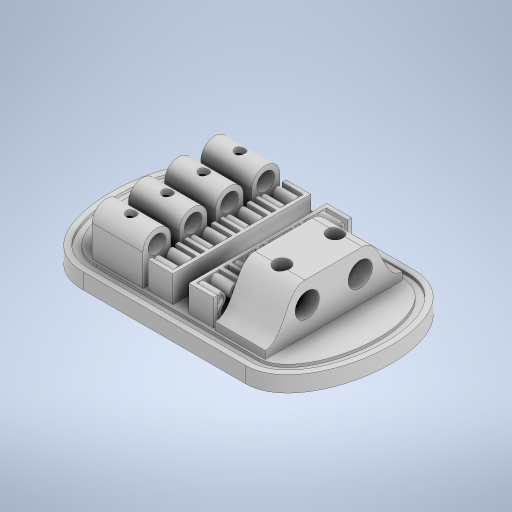
# Autodesk Inventor part: CO-1-01-fuseBox
Saved by Autodesk Inventor 2023 (Build 270158000, 158)
## iProperties
Created: 2023-02-27
Part Number: CO-1-01-fuseBox
Material: Generic
Document SubType Name: Modeling
Designer: t205b
Density: 1 g/cm^3
Appearance: Default
Author: t205b
Autodesk Inventor part; units mm, degrees
sketch "Sketch3" plane through (0, 0, 0) normal (0, 1, 0) x (-1, 0, 0)
  spline S0 degree 3 poles (-36.65, 37.75) (-66.3724, 37.75) (-73.5943, -37.75) (-36.65, -37.75) knots 0 0 0 0 1 1 1 1
  line L0 (-36.65, -37.75) -> (36.65, -37.75)
  line L1 (100, 0) -> (-100, 0)
  line L2 (0, 75) -> (0, -75)
  line L3 (140, 0) -> (-140, 0) projected
  line L4 (0, -105) -> (0, 105) projected
  line L5 (-36.65, 37.75) -> (36.65, 37.75)
  spline S1 degree 4 poles (36.65, 37.75) (64.3582, 37.75) (66.3724, 0) (64.3582, -37.75) (36.65, -37.75) knots 0 0 0 0 0 1 1 1 1 1
  point P0 (0, 0)
  point P1 (-61.65, 0)
  point P2 (0, 0)
  point P3 (61.65, 0)
  dimension "d32" = 200
  dimension "d33" = 150
  dimension "d34" = 75
  dimension "d35" = 100
  dimension "d36" = 37.75
  dimension "d37" = 61.65
  dimension "d38" = 25
  dimension "d39" = 75.5
  dimension "d40" = 25
  constraints: 8 end point, 6 horizontal, 2 collinear, 2 point on line, 2 symmetric about line, 1 midpoint, 1 vertical, 1 vertical alignment, 6 other
  measures "d32" distance of L1.start L1.end
  measures "d33" distance of L2.start L2.end
  measures "d34" distance of point (0, 0) L2.end
  measures "d35" distance of point (0, 0) L1.end
  measures "d36" distance between parallel lines of L1 L0
  measures "d37" distance from line of L2 point (-61.65, 0)
  measures "d38" horizontal distance of point (-61.65, 0) L0.start
  measures "d39" distance between parallel lines of L5 L0
  measures "d40" horizontal distance of L0.end point (61.65, 0)
extrude "Extrusion2" add sketch "Sketch3" along normal blind 7.2
sketch "Sketch4" plane through (0, 7.2, 0) normal (0, 1, 0) x (1, 0, 0)
  line L0 (-36.65, -37.75) -> (36.65, -37.75) projected
  spline S0 degree 3 poles (36.65, -37.75) (66.3724, -37.75) (73.5943, 37.75) (36.65, 37.75) knots 0 0 0 0 1 1 1 1
  line L1 (36.65, 37.75) -> (-36.65, 37.75) projected
  spline S1 degree 4 poles (-36.65, 37.75) (-64.3582, 37.75) (-66.3724, 0) (-64.3582, -37.75) (-36.65, -37.75) knots 0 0 0 0 0 1 1 1 1 1
  line L2 (36.65, -35.15) -> (-36.65, -35.15)
  line L3 (-36.65, 35.15) -> (36.65, 35.15)
  line L4 (36.65, -32) -> (-36.65, -32)
  line L5 (-36.65, 32) -> (36.65, 32)
  spline S2 degree 5 poles (-36.65, -35.15) (-38.7951, -35.149) (-40.9355, -34.9184) (-43.0555, -34.3853) (-46.9479, -32.645) (-50.1237, -29.806) (-51.4679, -28.2094) (-53.9958, -24.4798) (-55.7766, -20.3315) (-56.5612, -18.0325) (-57.9028, -13.0968) (-58.6606, -8.0384) (-58.9204, -5.3645) (-59.1796, 0) (-58.9204, 5.3645) (-58.6606, 8.0384) (-57.9028, 13.0968) (-56.5612, 18.0325) (-55.7766, 20.3315) (-53.9958, 24.4798) (-51.4679, 28.2094) (-50.1237, 29.806) (-46.9479, 32.645) (-43.0555, 34.3853) (-40.9355, 34.9184) (-38.7951, 35.149) (-36.65, 35.15) knots 0 0 0 0 0 0 0.11508 0.11508 0.11508 0.225967 0.225967 0.225967 0.356046 0.356046 0.356046 0.5 0.5 0.5 0.643954 0.643954 0.643954 0.774033 0.774033 0.774033 0.88492 0.88492 0.88492 1 1 1 1 1 1
  spline S3 degree 5 poles (36.65, 35.15) (38.8444, 35.1493) (41.0355, 34.9067) (43.1996, 34.3601) (47.1853, 32.6249) (50.4881, 29.804) (51.8967, 28.2119) (54.5079, 24.5102) (56.327, 20.3525) (57.1025, 18.0646) (58.3839, 13.1497) (59.0001, 8.107) (59.1641, 5.4459) (59.1963, 0.0809) (58.6482, -5.2565) (58.23, -7.9258) (57.1472, -13.0057) (55.486, -17.9261) (54.5457, -20.2359) (52.5203, -24.3703) (49.8538, -28.1181) (48.4863, -29.7243) (45.5873, -32.4365) (42.0779, -34.2692) (40.3126, -34.8729) (38.479, -35.1493) (36.65, -35.15) knots 0 0 0 0 0 0 0.118721 0.118721 0.118721 0.23255 0.23255 0.23255 0.362852 0.362852 0.362852 0.506829 0.506829 0.506829 0.652778 0.652778 0.652778 0.787419 0.787419 0.787419 0.900976 0.900976 0.900976 1 1 1 1 1 1
  spline S4 degree 5 poles (-36.65, -32) (-38.4313, -31.9991) (-40.2071, -31.8168) (-41.973, -31.3923) (-45.254, -29.9388) (-47.9096, -27.5288) (-49.0424, -26.1594) (-51.279, -22.8321) (-52.852, -19.1329) (-53.5716, -17.0114) (-54.8234, -12.3836) (-55.5313, -7.642) (-55.7772, -5.0998) (-56.0228, 0) (-55.7772, 5.0998) (-55.5313, 7.642) (-54.8234, 12.3836) (-53.5716, 17.0114) (-52.852, 19.1329) (-51.279, 22.8321) (-49.0424, 26.1594) (-47.9096, 27.5288) (-45.254, 29.9388) (-41.973, 31.3923) (-40.2071, 31.8168) (-38.4313, 31.9991) (-36.65, 32) knots 0 0 0 0 0 0 0.106905 0.106905 0.106905 0.21262 0.21262 0.21262 0.346882 0.346882 0.346882 0.5 0.5 0.5 0.653118 0.653118 0.653118 0.78738 0.78738 0.78738 0.893095 0.893095 0.893095 1 1 1 1 1 1
  spline S5 degree 5 poles (36.65, 32) (38.4906, 31.9993) (40.3274, 31.8039) (42.1467, 31.3587) (45.524, 29.8989) (48.3077, 27.4963) (49.5, 26.1293) (51.8011, 22.8434) (53.4009, 19.1536) (54.1048, 17.0615) (55.2895, 12.4921) (55.8589, 7.8049) (56.0122, 5.2946) (56.041, 0.221) (55.523, -4.8266) (55.127, -7.3572) (54.1106, -12.1313) (52.5533, -16.7561) (51.6809, -18.9069) (49.8554, -22.6513) (47.4533, -26.0492) (46.267, -27.4584) (43.8621, -29.7468) (40.9405, -31.2919) (39.5479, -31.7812) (38.0961, -31.9994) (36.65, -32) knots 0 0 0 0 0 0 0.111514 0.111514 0.111514 0.220328 0.220328 0.220328 0.353718 0.353718 0.353718 0.505824 0.505824 0.505824 0.66079 0.66079 0.66079 0.801131 0.801131 0.801131 0.912291 0.912291 0.912291 1 1 1 1 1 1
  point P0 (0, 0)
  dimension "d43" = 2.6
  dimension "d44" = 5.75
  constraints: 8 end point, 6 parallel, 6 vertical alignment, 8 other
  measures "d43" distance between parallel lines of L0 L2
  measures "d44" distance between parallel lines of L0 L4
ref_plane "Work Plane1" through (38.75, 0, 0) normal (1, 0, 0) x (0, 1, 0)
sketch "Sketch5" plane through (38.75, 0, 0) normal (1, 0, 0) x (0, 1, 0)
  line L0 (29.3, 13) -> (29.3, -13)
  line L1 (7.2, 31) -> (10.7, 31)
  line L2 (7.2, -31) -> (10.7, -31)
  line L3 (10.7, 31) -> (10.7, 22) construction
  line L4 (10.7, 22) -> (29.3, 22) construction
  line L5 (29.3, 22) -> (29.3, 13) construction
  spline S0 degree 3 poles (10.7, 31) (10.7, 22) (29.3, 22) (29.3, 13) knots 1 1 1 1 2 2 2 2
  line L6 (10.7, -31) -> (10.7, -22) construction
  line L7 (10.7, -22) -> (29.3, -22) construction
  line L8 (29.3, -22) -> (29.3, -13) construction
  spline S1 degree 3 poles (10.7, -31) (10.7, -22) (29.3, -22) (29.3, -13) knots 1 1 1 1 2 2 2 2
  line L9 (7.2, 31) -> (7.2, -31)
  line L10 (7.2, 37.75) -> (7.2, -37.75) projected
  line L11 (-6.2242, 0) -> (37.3454, 0) projected
  circle A0 centre (19.125, 12) radius 5.425
  circle A1 centre (19.125, -12) radius 5.425
  point P0 (0, 0)
  dimension "d46" = 22.1
  dimension "d47" = 62
  dimension "d48" = 31
  dimension "d49" = 3.5
  dimension "d51" = 26
  dimension "d52" = 13
  dimension "d53" = 10.85
  dimension "d54" = 12
  dimension "d55" = 12
  dimension "d56" = 10.175
  dimension "d57" = 10.175
  constraints: 8 end point, 6 vertical, 4 horizontal, 3 parallel, 2 centre point, 1 collinear, 1 equal radius, 6 other
  measures "d46" distance between parallel lines of L0 L9
  measures "d47" distance between parallel lines of L2 L1
  measures "d48" distance between parallel lines of L11 L2
  measures "d49" distance of L2.start L2.end
  measures "d51" distance of L0.start L0.end
  measures "d52" distance from line of L11 L0.end
  measures "d53" diameter of A1
  measures "d54" distance from line of L11 A1.centre
  measures "d55" distance from line of L11 A0.centre
  measures "d56" distance from line of L0 A1.centre
  measures "d57" distance from line of L0 A0.centre
extrude "Extrusion3" cut sketch "Sketch4" against normal blind 1.25 contours L2 S2 L3 S3
extrude "Extrusion4" add sketch "Sketch5" against normal blind 22.68
sketch "Sketch6" plane through (38.75, 29.3, 13) normal (0, 1, 0) x (1, 0, 0)
  line L0 (-22.68, -4.425) -> (-22.68, 6.425) projected
  line L1 (0, 6.425) -> (0, -4.425) projected
  line L2 (-22.68, 19.575) -> (-22.68, 30.425) projected
  line L3 (0, 30.425) -> (0, 19.575) projected
  line L4 (0, -18) -> (-22.68, -18) construction
  line L5 (-11.34, -18) -> (-11.34, 44) construction
  line L6 (-22.68, 44) -> (0, 44) construction
  line L7 (-22.68, -18) -> (-22.68, 44) construction
  line L8 (-22.68, 1) -> (0, 1) construction
  line L9 (0, 44) -> (0, -18) construction
  line L10 (-22.68, 25) -> (0, 25) construction
  circle A0 centre (-11.34, 1) radius 3.5
  circle A1 centre (-11.34, 25) radius 3.5
  point P0 (-38.75, 13)
  dimension "d62" = 7
  dimension "d63" = 7
  constraints: 7 midpoint, 6 end point, 3 point on line, 2 centre point, 1 perpendicular
  measures "d62" diameter of A0
  measures "d63" diameter of A1
extrude "Extrusion5" cut sketch "Sketch6" against normal blind 7
ref_plane "Work Plane2" through (-16.68, 0, 0) normal (-1, 0, 0) x (0, 0, 1)
sketch "Sketch7" plane through (-16.68, 0, 0) normal (-1, 0, 0) x (0, 0, 1)
  line L0 (-31, 10.7) -> (-31, 7.2) projected
  line L1 (-31, 7.2) -> (-31, 21.375)
  line L2 (-31, 7.2) -> (31, 7.2) projected
  line L3 (-18.35, 7.2) -> (-18.35, 21.375)
  arc A0 (-18.35, 21.375) -> (-31, 21.375) centre (-24.675, 21.375) ccw
  circle A1 centre (-24.675, 21.375) radius 4
  line L4 (-14.6, 7.2) -> (-14.6, 21.375)
  arc A2 (-1.95, 21.375) -> (-14.6, 21.375) centre (-8.275, 21.375) ccw
  circle A3 centre (-8.275, 21.375) radius 4
  line L5 (-1.95, 7.2) -> (-1.95, 21.375)
  line L6 (1.8, 7.2) -> (1.8, 21.375)
  arc A4 (14.45, 21.375) -> (1.8, 21.375) centre (8.125, 21.375) ccw
  circle A5 centre (8.125, 21.375) radius 4
  line L7 (14.45, 7.2) -> (14.45, 21.375)
  line L8 (18.2, 7.2) -> (18.2, 21.375)
  arc A6 (30.85, 21.375) -> (18.2, 21.375) centre (24.525, 21.375) ccw
  circle A7 centre (24.525, 21.375) radius 4
  line L9 (30.85, 7.2) -> (30.85, 21.375)
  point P0 (0, 0)
  point P1 (-31, 14.2875)
  point P2 (-14.6, 14.2875)
  point P3 (1.8, 14.2875)
  point P4 (18.2, 14.2875)
  dimension "d67" = 12.65
  dimension "d69" = 14.175
  dimension "d70" = 8
  dimension "d73" = 16.4
  constraints: 16 end point, 8 centre point, 8 point on circle, 4 coincident, 2 tangent, 2 vertical, 1 horizontal, 1 midpoint, 1 point on line, 33 other
  measures "d67" distance from line of point (-31, 14.288) L3
  measures "d69" distance from line of L2 A0.centre
  measures "d70" diameter of A1
  measures "d73" distance of L0.end L4.start
extrude "Extrusion6" add sketch "Sketch7" along normal blind 23
ref_plane "Work Plane3" through (0, 27.5, 0) normal (0, 1, 0) x (1, 0, 0)
sketch "Sketch8" plane through (0, 27.5, 0) normal (0, 1, 0) x (1, 0, 0)
  circle A0 centre (-28.23, 24.675) radius 2.2
  line L0 (-39.68, 20.675) -> (-39.68, 28.675) projected
  line L1 (-16.68, 18.35) -> (-39.68, 18.35) projected
  circle A1 centre (-28.23, 8.275) radius 2.2
  circle A2 centre (-28.23, -8.125) radius 2.2
  circle A3 centre (-28.23, -24.525) radius 2.2
  line L2 (-39.68, -28.525) -> (-39.68, -20.525) projected
  point P0 (0, 0)
  point P1 (-28.18, 18.35)
  dimension "d81" = 4.4
  dimension "d82" = 11.45
  dimension "d84" = 8
  dimension "d85" = 4
  dimension "d88" = 16.4
  constraints: 4 centre point, 1 midpoint, 1 vertical, 6 other
  measures "d81" diameter of A0
  measures "d82" distance from line of L0 A0.centre
  measures "d84" distance of L0.start L0.end
  measures "d85" vertical distance of A0.centre L0.start
  measures "d88" distance of A0.centre A1.centre
extrude "Extrusion7" cut sketch "Sketch8" along normal mid plane 6
sketch "Sketch9" plane through (0, 7.2, 0) normal (0, 1, 0) x (1, 0, 0)
  line L0 (14.87, -30.35) -> (3.62, -30.35)
  line L1 (3.62, -30.35) -> (3.62, 32.05)
  line L2 (3.62, 32.05) -> (14.87, 32.05)
  line L3 (36.65, 32) -> (-36.65, 32) projected
  line L4 (14.87, 32.05) -> (14.87, 30.25)
  line L5 (14.87, 30.25) -> (5.22, 30.25)
  line L6 (5.22, 30.25) -> (5.22, 19.75)
  line L7 (5.22, 19.75) -> (14.87, 19.75)
  line L8 (14.87, 19.75) -> (14.87, 17.95)
  line L9 (14.87, 17.95) -> (5.22, 17.95)
  line L10 (5.22, 17.95) -> (5.22, 15.95)
  line L11 (5.22, 15.95) -> (14.87, 15.95)
  line L12 (14.87, 15.95) -> (14.87, 14.15)
  line L13 (14.87, 14.15) -> (5.22, 14.15)
  line L14 (5.22, 14.15) -> (5.22, 3.65)
  line L15 (5.22, 3.65) -> (14.87, 3.65)
  line L16 (14.87, 3.65) -> (14.87, 1.85)
  line L17 (14.87, 1.85) -> (5.22, 1.85)
  line L18 (5.22, 1.85) -> (5.22, -0.15)
  line L19 (5.22, -0.15) -> (14.87, -0.15)
  line L20 (14.87, -0.15) -> (14.87, -1.95)
  line L21 (14.87, -1.95) -> (5.22, -1.95)
  line L22 (5.22, -1.95) -> (5.22, -12.45)
  line L23 (5.22, -12.45) -> (14.87, -12.45)
  line L24 (14.87, -12.45) -> (14.87, -14.25)
  line L25 (14.87, -14.25) -> (5.22, -14.25)
  line L26 (14.87, -30.35) -> (14.87, -28.55)
  line L27 (14.87, -28.55) -> (5.22, -28.55)
  line L28 (5.22, -28.55) -> (5.22, -18.05)
  line L29 (5.22, -18.05) -> (14.87, -18.05)
  line L30 (14.87, -18.05) -> (14.87, -16.25)
  line L31 (14.87, -16.25) -> (5.22, -16.25)
  line L32 (5.22, -16.25) -> (5.22, -14.25)
  line L33 (-36.65, -37.75) -> (36.65, -37.75) projected
  line L34 (16.07, -31) -> (16.07, 31) projected
  point P0 (0, 0)
  dimension "d96" = 1.8
  dimension "d97" = 10.5
  dimension "d99" = 2
  dimension "d100" = 7.4
  dimension "d101" = 1.2
  dimension "d102" = 11.25
  dimension "d103" = 1.6
  dimension "d104" = 9.65
  constraints: 64 end point, 21 perpendicular, 15 equal length, 15 point on line, 3 vertical, 1 horizontal, 1 parallel
  measures "d96" distance of L2.end L4.end
  measures "d97" distance of L5.end L6.end
  measures "d99" distance of L9.end L10.end
  measures "d100" distance between parallel lines of L0 L33
  measures "d101" distance between parallel lines of L34 L26
  measures "d102" distance of L0.start L0.end
  measures "d103" distance between parallel lines of L1 L28
  measures "d104" distance of L28.end L29.end
extrude "Extrusion8" add sketch "Sketch9" along normal blind 12
mirror "Mirror1" about plane through (0, 0, 0) normal (1, 0, 0) of "Extrusion8"
sketch "Sketch10" plane through (5.22, 7.2, -19.75) normal (1, 0, 0) x (0, 0, -1)
  spline S0 degree 4 poles (9.425, 7.8) (9.2346, 15.5874) (3.5799, 6.3679) (8.4396, 8.6805) (9.5353, 0.0883) (0.3147, 0.0883) (1.4104, 8.6805) (6.2701, 6.3679) (0.6154, 15.5874) (0.425, 7.8) knots 0 0 0 0 0 0.26738 0.381915 0.5 0.618085 0.73262 1 1 1 1 1
  line L0 (18, -7.2) -> (-57.5, -7.2) projected
  circle A0 centre (4.925, 14.175) radius 4 projected
  line L1 (10.5, 0) -> (10.5, 12) projected
  line L2 (0, 0) -> (0, 12) projected
  spline S1 degree 5 poles (9.9249, 7.8122) (9.9112, 8.3424) (9.8831, 8.8754) (9.8254, 9.4003) (9.6956, 10.2438) (9.3803, 11.0296) (9.233, 11.3105) (8.8447, 11.7572) (8.2849, 11.9289) (8.0172, 11.9254) (7.5499, 11.7927) (7.1572, 11.5101) (6.9913, 11.3552) (6.6866, 11.0187) (6.4376, 10.6387) (6.3248, 10.4411) (6.1283, 10.0415) (5.9805, 9.6217) (5.9206, 9.4124) (5.832, 9.0043) (5.8023, 8.5879) (5.8032, 8.3877) (5.8388, 8.0043) (5.9426, 7.634) (6.0089, 7.4611) (6.1664, 7.143) (6.3707, 6.853) (6.4774, 6.7205) (6.6955, 6.473) (6.9228, 6.2339) (7.0324, 6.1174) (7.2492, 5.8753) (7.4479, 5.6181) (7.5423, 5.4826) (7.7229, 5.1905) (7.8675, 4.8789) (7.9319, 4.7123) (8.0408, 4.3629) (8.0994, 4.0015) (8.1154, 3.8144) (8.1173, 3.4409) (8.0532, 3.0731) (8.0035, 2.8936) (7.8624, 2.5396) (7.6466, 2.2251) (7.518, 2.0776) (7.2077, 1.7895) (6.8448, 1.5698) (6.6387, 1.4707) (6.1823, 1.2955) (5.7036, 1.1939) (5.4451, 1.1586) (4.925, 1.1234) (4.4049, 1.1586) (4.1464, 1.1939) (3.6677, 1.2955) (3.2113, 1.4707) (3.0052, 1.5698) (2.6423, 1.7895) (2.332, 2.0776) (2.2034, 2.2251) (1.9876, 2.5396) (1.8465, 2.8936) (1.7968, 3.0731) (1.7327, 3.4409) (1.7346, 3.8144) (1.7506, 4.0015) (1.8092, 4.3629) (1.9181, 4.7123) (1.9825, 4.8789) (2.1271, 5.1905) (2.3077, 5.4826) (2.4021, 5.6181) (2.6008, 5.8753) (2.8176, 6.1174) (2.9272, 6.2339) (3.1545, 6.473) (3.3726, 6.7205) (3.4793, 6.853) (3.6836, 7.143) (3.8411, 7.4611) (3.9074, 7.634) (4.0112, 8.0043) (4.0468, 8.3877) (4.0477, 8.5879) (4.018, 9.0043) (3.9294, 9.4124) (3.8695, 9.6217) (3.7217, 10.0415) (3.5252, 10.4411) (3.4124, 10.6387) (3.1634, 11.0187) (2.8587, 11.3552) (2.6928, 11.5101) (2.3001, 11.7927) (1.8328, 11.9254) (1.5651, 11.9289) (1.0053, 11.7572) (0.617, 11.3105) (0.4697, 11.0296) (0.1544, 10.2438) (0.0246, 9.4003) (-0.0331, 8.8754) (-0.0612, 8.3424) (-0.0749, 7.8122) knots 0 0 0 0 0 0 0.068516 0.068516 0.068516 0.108925 0.108925 0.108925 0.141412 0.141412 0.141412 0.170512 0.170512 0.170512 0.199827 0.199827 0.199827 0.227844 0.227844 0.227844 0.253557 0.253557 0.253557 0.277287 0.277287 0.277287 0.299199 0.299199 0.299199 0.31984 0.31984 0.31984 0.341106 0.341106 0.341106 0.364074 0.364074 0.364074 0.388214 0.388214 0.388214 0.412061 0.412061 0.412061 0.437092 0.437092 0.437092 0.466447 0.466447 0.466447 0.5 0.5 0.5 0.533553 0.533553 0.533553 0.562908 0.562908 0.562908 0.587939 0.587939 0.587939 0.611786 0.611786 0.611786 0.635926 0.635926 0.635926 0.658894 0.658894 0.658894 0.68016 0.68016 0.68016 0.700801 0.700801 0.700801 0.722713 0.722713 0.722713 0.746443 0.746443 0.746443 0.772156 0.772156 0.772156 0.800173 0.800173 0.800173 0.829488 0.829488 0.829488 0.858588 0.858588 0.858588 0.891075 0.891075 0.891075 0.931484 0.931484 0.931484 1 1 1 1 1 1
  spline S2 degree 5 poles (8.9251, 7.7878) (8.9156, 8.1863) (8.8951, 8.5845) (8.862, 8.982) (8.7864, 9.5781) (8.6369, 10.1595) (8.5726, 10.3494) (8.4781, 10.5939) (8.3163, 10.7986) (8.2781, 10.8377) (8.1878, 10.9138) (8.0751, 10.8858) (8.0329, 10.8704) (7.8948, 10.8043) (7.7769, 10.7091) (7.7001, 10.6385) (7.5384, 10.4662) (7.3981, 10.2754) (7.3256, 10.1643) (7.1896, 9.9331) (7.076, 9.6902) (7.0241, 9.565) (6.9367, 9.3229) (6.8726, 9.0735) (6.848, 8.9541) (6.8146, 8.7326) (6.8071, 8.5088) (6.8097, 8.4067) (6.8275, 8.2172) (6.872, 8.0324) (6.8987, 7.9482) (6.9658, 7.7815) (7.0552, 7.6255) (7.1058, 7.5492) (7.2257, 7.386) (7.3586, 7.233) (7.4336, 7.1511) (7.6023, 6.9707) (7.7708, 6.7903) (7.8622, 6.6896) (8.0538, 6.4687) (8.2324, 6.2371) (8.3234, 6.1097) (8.5042, 5.834) (8.6602, 5.5436) (8.7347, 5.3872) (8.8735, 5.0555) (8.9774, 4.7111) (9.0214, 4.5298) (9.0913, 4.1524) (9.1162, 3.7693) (9.1167, 3.5718) (9.091, 3.1693) (9.0079, 2.7746) (8.9499, 2.5766) (8.7993, 2.1842) (8.5857, 1.8222) (8.4611, 1.6475) (8.1767, 1.3127) (7.8413, 1.0287) (7.6582, 0.8975) (7.2631, 0.6563) (6.8378, 0.4729) (6.6134, 0.3934) (6.1464, 0.2593) (5.6669, 0.1807) (5.4202, 0.1542) (4.925, 0.1278) (4.4298, 0.1542) (4.1831, 0.1807) (3.7036, 0.2593) (3.2366, 0.3934) (3.0122, 0.4729) (2.5869, 0.6563) (2.1918, 0.8975) (2.0087, 1.0287) (1.6733, 1.3127) (1.3889, 1.6475) (1.2643, 1.8222) (1.0507, 2.1842) (0.9001, 2.5766) (0.8421, 2.7746) (0.759, 3.1693) (0.7333, 3.5718) (0.7338, 3.7693) (0.7587, 4.1524) (0.8286, 4.5298) (0.8726, 4.7111) (0.9765, 5.0555) (1.1153, 5.3872) (1.1898, 5.5436) (1.3458, 5.834) (1.5266, 6.1097) (1.6176, 6.2371) (1.7962, 6.4687) (1.9878, 6.6896) (2.0792, 6.7903) (2.2477, 6.9707) (2.4164, 7.1511) (2.4914, 7.233) (2.6243, 7.386) (2.7442, 7.5492) (2.7948, 7.6255) (2.8842, 7.7815) (2.9513, 7.9482) (2.978, 8.0324) (3.0225, 8.2172) (3.0403, 8.4067) (3.0429, 8.5088) (3.0354, 8.7326) (3.002, 8.9541) (2.9774, 9.0735) (2.9133, 9.3229) (2.8259, 9.565) (2.774, 9.6902) (2.6604, 9.9331) (2.5244, 10.1643) (2.4519, 10.2754) (2.3116, 10.4662) (2.1499, 10.6385) (2.0731, 10.7091) (1.9552, 10.8043) (1.8171, 10.8704) (1.7749, 10.8858) (1.6622, 10.9138) (1.5719, 10.8377) (1.5337, 10.7986) (1.3719, 10.5939) (1.2774, 10.3494) (1.2131, 10.1595) (1.0636, 9.5781) (0.988, 8.982) (0.9549, 8.5845) (0.9344, 8.1863) (0.9249, 7.7878) knots 0 0 0 0 0 0 0.055885 0.055885 0.055885 0.084022 0.084022 0.084022 0.092088 0.092088 0.092088 0.098739 0.098739 0.098739 0.11327 0.11327 0.11327 0.131845 0.131845 0.131845 0.150825 0.150825 0.150825 0.167895 0.167895 0.167895 0.182171 0.182171 0.182171 0.194496 0.194496 0.194496 0.207309 0.207309 0.207309 0.222875 0.222875 0.222875 0.241932 0.241932 0.241932 0.263859 0.263859 0.263859 0.288106 0.288106 0.288106 0.314213 0.314213 0.314213 0.341823 0.341823 0.341823 0.370614 0.370614 0.370614 0.400541 0.400541 0.400541 0.431996 0.431996 0.431996 0.465289 0.465289 0.465289 0.5 0.5 0.5 0.534711 0.534711 0.534711 0.568004 0.568004 0.568004 0.599459 0.599459 0.599459 0.629386 0.629386 0.629386 0.658177 0.658177 0.658177 0.685787 0.685787 0.685787 0.711894 0.711894 0.711894 0.736141 0.736141 0.736141 0.758068 0.758068 0.758068 0.777125 0.777125 0.777125 0.792691 0.792691 0.792691 0.805504 0.805504 0.805504 0.817829 0.817829 0.817829 0.832105 0.832105 0.832105 0.849175 0.849175 0.849175 0.868155 0.868155 0.868155 0.88673 0.88673 0.88673 0.901261 0.901261 0.901261 0.907912 0.907912 0.907912 0.915978 0.915978 0.915978 0.944115 0.944115 0.944115 1 1 1 1 1 1
  point P0 (-19.75, -7.2)
  point P1 (7.175, 10.8)
  point P2 (6.425, 7.8)
  point P3 (7.925, 5.8)
  point P4 (7.925, 1.8)
  point P5 (1.925, 1.8)
  point P6 (1.925, 5.8)
  point P7 (3.425, 7.8)
  point P8 (2.675, 10.8)
  dimension "d145" = 0.5
  dimension "d146" = 0.5
  dimension "d107" = 9
  dimension "d108" = 3
  dimension "d109" = 6
  dimension "d110" = 3
  dimension "d111" = 1.5
  dimension "d113" = 4.5
  dimension "d114" = 6
  dimension "d115" = 3
  dimension "d116" = 4.5
  dimension "d117" = 2.25
  dimension "d128" = 9
  dimension "d131" = 3
  dimension "d132" = 2
  dimension "d134" = 9
  constraints: 8 horizontal alignment, 14 other
  measures "d107" distance from line of point (7.925, 1.8) L0
  measures "d108" distance of point (6.425, 7.8) point (3.425, 7.8)
  measures "d109" distance of point (1.925, 5.8) point (7.925, 5.8)
  measures "d110" horizontal distance of point (7.925, 5.8) A0.centre
  measures "d111" horizontal distance of A0.centre point (6.425, 7.8)
  measures "d113" horizontal distance of point (9.425, 7.8) A0.centre
  measures "d114" distance of point (1.925, 1.8) point (7.925, 1.8)
  measures "d115" horizontal distance of point (7.925, 1.8) A0.centre
  measures "d116" distance of point (2.675, 10.8) point (7.175, 10.8)
  measures "d117" horizontal distance of point (7.175, 10.8) A0.centre
  measures "d128" vertical distance of point (7.175, 10.8) point (7.925, 1.8)
  measures "d131" vertical distance of point (9.425, 7.8) point (7.175, 10.8)
  measures "d132" vertical distance of point (6.425, 7.8) point (7.925, 5.8)
  measures "d134" distance of point (0.425, 7.8) point (9.425, 7.8)
sketch "Sketch11" plane through (5.22, 7.2, -19.75) normal (1, 0, 0) x (0, 0, -1)
  spline S0 degree 3 poles (8.9251, 7.7878) (8.9155, 8.182) (8.8741, 8.8814) (8.7781, 9.5528) (8.671, 10.0317) (8.591, 10.2839) (8.5088, 10.4858) (8.454, 10.5957) (8.3882, 10.7043) (8.3392, 10.7691) (8.2908, 10.8204) (8.2632, 10.8441) (8.2394, 10.8612) (8.2254, 10.8698) (8.21, 10.8778) (8.1991, 10.8824) (8.1867, 10.8866) (8.1774, 10.889) (8.1656, 10.891) (8.1557, 10.892) (8.1421, 10.8924) (8.13, 10.8919) (8.1093, 10.8895) (8.0851, 10.8848) (8.0419, 10.8717) (7.9966, 10.8526) (7.9205, 10.8115) (7.8352, 10.7535) (7.6994, 10.6366) (7.5755, 10.5043) (7.4257, 10.3122) (7.3122, 10.1409) (7.1833, 9.9132) (7.0917, 9.7231) (6.9941, 9.4824) (6.9303, 9.2898) (6.8694, 9.0545) (6.8358, 8.8724) (6.8124, 8.656) (6.8083, 8.4929) (6.8198, 8.3029) (6.8418, 8.1619) (6.8838, 7.9974) (6.9286, 7.8738) (6.9989, 7.7251) (7.0671, 7.6091) (7.1886, 7.4344) (7.3365, 7.2561) (7.6068, 6.9651) (7.8875, 6.6675) (8.2098, 6.2718) (8.4177, 5.971) (8.6086, 5.6398) (8.7255, 5.4039) (8.8546, 5.0912) (8.9426, 4.8274) (9.0294, 4.4828) (9.0789, 4.1963) (9.1117, 3.8278) (9.113, 3.5263) (9.0789, 3.1453) (9.0211, 2.8396) (8.9069, 2.4636) (8.7812, 2.1705) (8.5805, 1.821) (8.3855, 1.5576) (8.1014, 1.2546) (7.8436, 1.0351) (7.4877, 0.7924) (7.1781, 0.6245) (6.7655, 0.449) (6.417, 0.3363) (5.9641, 0.2305) (5.5906, 0.174) (5.1162, 0.1387) (4.7338, 0.1387) (4.2594, 0.174) (3.8859, 0.2305) (3.433, 0.3363) (3.0845, 0.449) (2.6719, 0.6245) (2.3623, 0.7924) (2.0064, 1.0351) (1.7486, 1.2546) (1.4645, 1.5576) (1.2695, 1.821) (1.0688, 2.1705) (0.9431, 2.4636) (0.8289, 2.8396) (0.7711, 3.1453) (0.737, 3.5263) (0.7383, 3.8278) (0.7711, 4.1963) (0.8206, 4.4828) (0.9074, 4.8274) (0.9954, 5.0912) (1.1245, 5.4039) (1.2414, 5.6398) (1.4323, 5.971) (1.6402, 6.2718) (1.9625, 6.6675) (2.2432, 6.9651) (2.5135, 7.2561) (2.6614, 7.4344) (2.7829, 7.6091) (2.8511, 7.7251) (2.9214, 7.8738) (2.9662, 7.9974) (3.0082, 8.1619) (3.0302, 8.3029) (3.0417, 8.4929) (3.0376, 8.656) (3.0142, 8.8724) (2.9806, 9.0545) (2.9197, 9.2898) (2.8559, 9.4824) (2.7583, 9.7231) (2.6667, 9.9132) (2.5378, 10.1409) (2.4243, 10.3122) (2.2745, 10.5043) (2.1506, 10.6366) (2.0148, 10.7535) (1.9295, 10.8115) (1.8534, 10.8526) (1.8081, 10.8717) (1.7649, 10.8848) (1.7407, 10.8895) (1.72, 10.8919) (1.7079, 10.8924) (1.6943, 10.892) (1.6844, 10.891) (1.6726, 10.889) (1.6633, 10.8866) (1.6509, 10.8824) (1.64, 10.8778) (1.6246, 10.8698) (1.6106, 10.8612) (1.5868, 10.8441) (1.5592, 10.8204) (1.5108, 10.7691) (1.4618, 10.7043) (1.396, 10.5957) (1.3412, 10.4858) (1.259, 10.2839) (1.179, 10.0317) (1.0719, 9.5528) (0.9759, 8.8814) (0.9345, 8.182) (0.9249, 7.7878) knots 0 0 0 0 0.010417 0.020833 0.026042 0.033854 0.036458 0.041667 0.044271 0.049479 0.052083 0.05599 0.057292 0.059896 0.061198 0.063802 0.065104 0.067708 0.06901 0.071615 0.072917 0.075521 0.076823 0.080729 0.083333 0.088542 0.091146 0.098958 0.104167 0.114583 0.119792 0.130208 0.135417 0.145833 0.151042 0.161458 0.166667 0.177083 0.182292 0.192708 0.197917 0.208333 0.213542 0.223958 0.229167 0.239583 0.244792 0.260417 0.270833 0.291667 0.302083 0.317708 0.322917 0.333333 0.338542 0.348958 0.354167 0.364583 0.369792 0.380208 0.385417 0.395833 0.401042 0.411458 0.416667 0.427083 0.432292 0.442708 0.447917 0.458333 0.463542 0.473958 0.479167 0.489583 0.494792 0.505208 0.510417 0.520833 0.526042 0.536458 0.541667 0.552083 0.557292 0.567708 0.572917 0.583333 0.588542 0.598958 0.604167 0.614583 0.619792 0.630208 0.635417 0.645833 0.651042 0.661458 0.666667 0.677083 0.682292 0.697917 0.708333 0.729167 0.739583 0.755208 0.760417 0.770833 0.776042 0.786458 0.791667 0.802083 0.807292 0.817708 0.822917 0.833333 0.838542 0.848958 0.854167 0.864583 0.869792 0.880208 0.885417 0.895833 0.901042 0.908854 0.911458 0.916667 0.919271 0.923177 0.924479 0.927083 0.928385 0.93099 0.932292 0.934896 0.936198 0.938802 0.940104 0.942708 0.94401 0.947917 0.950521 0.955729 0.958333 0.963542 0.966146 0.973958 0.979167 0.989583 1 1 1 1 projected
  spline S1 degree 3 poles (9.9249, 7.8122) (9.9147, 8.227) (9.8709, 8.9728) (9.7651, 9.721) (9.6387, 10.2877) (9.5374, 10.6112) (9.4213, 10.8969) (9.3362, 11.0693) (9.2187, 11.2641) (9.115, 11.4036) (8.9715, 11.5573) (8.845, 11.6628) (8.6901, 11.7587) (8.5809, 11.8089) (8.4686, 11.8471) (8.3927, 11.8665) (8.2975, 11.8833) (8.2214, 11.8908) (8.1273, 11.8932) (8.0532, 11.8897) (7.9444, 11.8773) (7.8391, 11.8557) (7.6887, 11.8094) (7.5631, 11.7553) (7.3857, 11.6592) (7.2219, 11.5455) (6.9964, 11.3508) (6.8152, 11.1555) (6.5679, 10.8385) (6.353, 10.4942) (6.1201, 10.011) (5.9878, 9.6394) (5.8917, 9.2687) (5.8462, 9.0231) (5.8134, 8.7205) (5.807, 8.4826) (5.8245, 8.1927) (5.8591, 7.9678) (5.9278, 7.698) (6.0024, 7.4925) (6.1169, 7.2509) (6.2235, 7.0703) (6.3699, 6.8601) (6.4952, 6.7036) (6.6565, 6.5189) (6.7871, 6.3783) (6.9483, 6.206) (7.0753, 6.0683) (7.2298, 5.8913) (7.3494, 5.7443) (7.492, 5.5507) (7.5999, 5.3872) (7.7248, 5.1705) (7.8156, 4.9871) (7.9154, 4.7454) (7.983, 4.5426) (8.0493, 4.2793) (8.0868, 4.062) (8.1113, 3.7857) (8.1121, 3.5629) (8.0874, 3.2878) (8.0465, 3.0724) (7.9675, 2.8125) (7.8818, 2.6128) (7.7454, 2.3754) (7.6124, 2.1956) (7.4151, 1.985) (7.2322, 1.8288) (6.9721, 1.6514) (6.7396, 1.5249) (6.421, 1.3893) (6.1454, 1.2999) (5.7805, 1.2146) (5.4749, 1.1682) (5.0835, 1.1391) (4.7665, 1.1391) (4.3751, 1.1682) (4.0695, 1.2146) (3.7046, 1.2999) (3.429, 1.3893) (3.1104, 1.5249) (2.8779, 1.6514) (2.6178, 1.8288) (2.4349, 1.985) (2.2376, 2.1956) (2.1046, 2.3754) (1.9682, 2.6128) (1.8825, 2.8125) (1.8035, 3.0724) (1.7626, 3.2878) (1.7379, 3.5629) (1.7387, 3.7857) (1.7632, 4.062) (1.8007, 4.2793) (1.867, 4.5426) (1.9346, 4.7454) (2.0344, 4.9871) (2.1252, 5.1705) (2.2501, 5.3872) (2.358, 5.5507) (2.5006, 5.7443) (2.6202, 5.8913) (2.7747, 6.0683) (2.9017, 6.206) (3.0629, 6.3783) (3.1935, 6.5189) (3.3548, 6.7036) (3.4801, 6.8601) (3.6265, 7.0703) (3.7331, 7.2509) (3.8476, 7.4925) (3.9222, 7.698) (3.9909, 7.9678) (4.0255, 8.1927) (4.043, 8.4826) (4.0366, 8.7205) (4.0038, 9.0231) (3.9583, 9.2687) (3.8622, 9.6394) (3.7299, 10.011) (3.497, 10.4942) (3.2821, 10.8385) (3.0348, 11.1555) (2.8536, 11.3508) (2.6281, 11.5455) (2.4643, 11.6592) (2.2869, 11.7553) (2.1613, 11.8094) (2.0109, 11.8557) (1.9056, 11.8773) (1.7968, 11.8897) (1.7227, 11.8932) (1.6286, 11.8908) (1.5525, 11.8833) (1.4573, 11.8665) (1.3814, 11.8471) (1.2691, 11.8089) (1.1599, 11.7587) (1.005, 11.6628) (0.8785, 11.5573) (0.735, 11.4036) (0.6313, 11.2641) (0.5138, 11.0693) (0.4287, 10.8969) (0.3126, 10.6112) (0.2113, 10.2877) (0.0849, 9.721) (-0.0209, 8.9728) (-0.0647, 8.227) (-0.0749, 7.8122) knots 0 0 0 0 0.010417 0.020833 0.026042 0.033854 0.036458 0.041667 0.044271 0.049479 0.052083 0.057292 0.059896 0.063802 0.065104 0.067708 0.06901 0.071615 0.072917 0.075521 0.076823 0.080729 0.083333 0.088542 0.091146 0.098958 0.104167 0.114583 0.119792 0.135417 0.145833 0.161458 0.166667 0.177083 0.182292 0.192708 0.197917 0.208333 0.213542 0.223958 0.229167 0.239583 0.244792 0.255208 0.260417 0.270833 0.276042 0.286458 0.291667 0.302083 0.307292 0.317708 0.322917 0.333333 0.338542 0.348958 0.354167 0.364583 0.369792 0.380208 0.385417 0.395833 0.401042 0.411458 0.416667 0.427083 0.432292 0.442708 0.447917 0.458333 0.463542 0.473958 0.479167 0.489583 0.494792 0.505208 0.510417 0.520833 0.526042 0.536458 0.541667 0.552083 0.557292 0.567708 0.572917 0.583333 0.588542 0.598958 0.604167 0.614583 0.619792 0.630208 0.635417 0.645833 0.651042 0.661458 0.666667 0.677083 0.682292 0.692708 0.697917 0.708333 0.713542 0.723958 0.729167 0.739583 0.744792 0.755208 0.760417 0.770833 0.776042 0.786458 0.791667 0.802083 0.807292 0.817708 0.822917 0.833333 0.838542 0.854167 0.864583 0.880208 0.885417 0.895833 0.901042 0.908854 0.911458 0.916667 0.919271 0.923177 0.924479 0.927083 0.928385 0.93099 0.932292 0.934896 0.936198 0.940104 0.942708 0.947917 0.950521 0.955729 0.958333 0.963542 0.966146 0.973958 0.979167 0.989583 1 1 1 1 projected
  line L0 (0, 0) -> (0, 12) projected
  line L1 (-0.0749, 7.8122) -> (0.9249, 7.7878)
  line L2 (8.9251, 7.7878) -> (9.9249, 7.8122)
  point P0 (-19.75, -7.2)
  point P1 (0, 9.0427)
  point P2 (0, 7.8104)
  constraints: 4 end point
extrude "Extrusion9" add sketch "Sketch11" along normal blind 9 contours S0 L1 L0 S1 L2
pattern_linear "Rectangular Pattern1" count 4 spacing 16 along (0, 0, 1) count 2 spacing 19.75 along (-1, 0, 0) of "Extrusion9"
body "Solid2"
